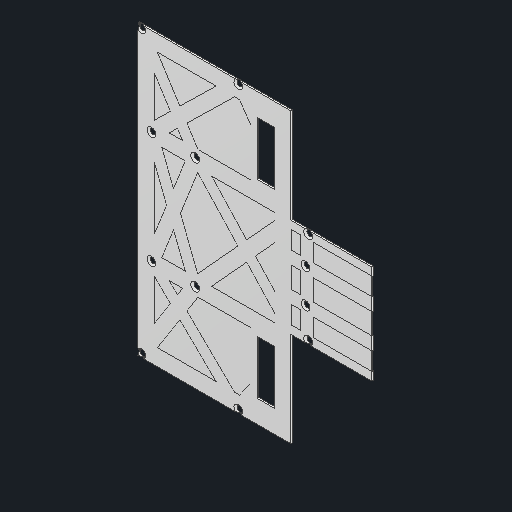
# Autodesk Inventor part: ceil
Saved by Autodesk Inventor 2023 (Build 270158000, 158)
## iProperties
Created: 2024-05-20
Part Number: ceil
Material: ABS Plastic
Document SubType Name: Modeling
Designer: szymo
Density: 1.06 g/cm^3
Appearance: Smooth - White
Mass: 13.9747 g
Surface Area: 401.437 cm^2
Volume: 13.1837 cm^3
Author: szymo
Autodesk Inventor part; units mm, degrees
ref_plane "YZ Plane" through (0, 0, 0) normal (1, 0, 0) x (0, 1, 0)
ref_plane "XZ Plane" through (0, 0, 0) normal (0, 1, 0) x (-1, 0, 0)
ref_plane "XY Plane" through (0, 0, 0) normal (0, 0, 1) x (1, 0, 0)
sketch "Sketch1" plane through (0, 0, 0) normal (0, 0, 1) x (1, 0, 0)
  arc A0 (-30.366, -174.5) -> (-31.2321, -174) centre (-31.2321, -175) ccw
  line L0 (-31.2321, -174) -> (-33.7679, -174)
  arc A1 (-33.7679, -174) -> (-34.634, -174.5) centre (-33.7679, -175) ccw
  arc A2 (-35.5, -175) -> (-34.634, -174.5) centre (-35.5, -174) ccw
  line L1 (-35.5, -175) -> (-89.4385, -175)
  arc A3 (-90.3045, -174.5) -> (-89.4385, -175) centre (-89.4385, -174) ccw
  arc A4 (-90.3045, -174.5) -> (-91.1706, -174) centre (-91.1706, -175) ccw
  line L2 (-91.1706, -174) -> (-93.7065, -174)
  arc A5 (-93.7065, -174) -> (-94.4385, -174.3187) centre (-93.7065, -175) ccw
  line L3 (-94.4385, -178) -> (-94.4385, -174.3187)
  line L4 (-94.4385, -178) -> (0, -178)
  line L5 (0, -178) -> (0, -175)
  line L6 (0, -175) -> (-29.5, -175)
  arc A6 (-30.366, -174.5) -> (-29.5, -175) centre (-29.5, -174) ccw
  circle A7 centre (-92.4385, -176) radius 1.75
  circle A8 centre (-32.5, -176) radius 1.75
  arc A9 (-31.2321, -4) -> (-30.366, -3.5) centre (-31.2321, -3) ccw
  arc A10 (-29.5, -3) -> (-30.366, -3.5) centre (-29.5, -4) ccw
  line L7 (0, -3) -> (-29.5, -3)
  line L8 (0, 0) -> (0, -3)
  line L9 (-94.4385, 0) -> (0, 0)
  line L10 (-94.4385, 0) -> (-94.4385, -3.6813)
  arc A11 (-94.4385, -3.6813) -> (-93.7065, -4) centre (-93.7065, -3) ccw
  line L11 (-91.1706, -4) -> (-93.7065, -4)
  arc A12 (-91.1706, -4) -> (-90.3045, -3.5) centre (-91.1706, -3) ccw
  arc A13 (-89.4385, -3) -> (-90.3045, -3.5) centre (-89.4385, -4) ccw
  line L12 (-35.5, -3) -> (-89.4385, -3)
  arc A14 (-34.634, -3.5) -> (-35.5, -3) centre (-35.5, -4) ccw
  arc A15 (-34.634, -3.5) -> (-33.7679, -4) centre (-33.7679, -3) ccw
  line L13 (-31.2321, -4) -> (-33.7679, -4)
  circle A16 centre (-92.4385, -2) radius 1.75
  circle A17 centre (-32.5, -2) radius 1.75
  circle A18 centre (-59.1371, -54.5) radius 1.75
  circle A19 centre (-86.1669, -54.5) radius 1.75
  spline S0 degree 2 poles (-1.1972, -52) (-3, -52.9286) (-4.8028, -52) knots 0 0 0 1 1 1 weights 1 1.166667 1
  line L14 (-25.1972, -52) -> (-4.8028, -52)
  spline S1 degree 2 poles (-25.1972, -52) (-27, -52.9286) (-28.8028, -52) knots 0 0 0 1 1 1 weights 1 1.166667 1
  line L15 (-94.4385, -52) -> (-28.8028, -52)
  line L16 (-94.4385, -52) -> (-94.4385, -57)
  line L17 (0, -57) -> (-94.4385, -57)
  line L18 (0, -52) -> (0, -57)
  line L19 (-1.1972, -52) -> (0, -52)
  circle A20 centre (-59.1371, -123.5) radius 1.75
  circle A21 centre (-86.1669, -123.5) radius 1.75
  spline S2 degree 2 poles (-1.1972, -126) (-3, -125.0714) (-4.8028, -126) knots 0 0 0 1 1 1 weights 1 1.166667 1
  line L20 (-1.1972, -126) -> (0, -126)
  line L21 (0, -126) -> (0, -121)
  line L22 (0, -121) -> (-94.4385, -121)
  line L23 (-94.4385, -126) -> (-94.4385, -121)
  line L24 (-94.4385, -126) -> (-28.8028, -126)
  spline S3 degree 2 poles (-25.1972, -126) (-27, -125.0714) (-28.8028, -126) knots 0 0 0 1 1 1 weights 1 1.166667 1
  line L25 (-25.1972, -126) -> (-4.8028, -126)
  circle A22 centre (10.6679, -117.5) radius 1.75
  arc A23 (45.504, -115.5) -> (44.7587, -115.8333) centre (45.504, -116.5) ccw
  arc A24 (43.2679, -116.5) -> (44.7587, -115.8333) centre (43.2679, -114.5) ccw
  line L26 (43.2679, -116.5) -> (13.6679, -116.5)
  arc A25 (12.8019, -116) -> (13.6679, -116.5) centre (13.6679, -115.5) ccw
  arc A26 (12.8019, -116) -> (11.9359, -115.5) centre (11.9359, -116.5) ccw
  line L27 (9.4, -115.5) -> (11.9359, -115.5)
  arc A27 (9.4, -115.5) -> (8.534, -116) centre (9.4, -116.5) ccw
  arc A28 (7.6679, -116.5) -> (8.534, -116) centre (7.6679, -115.5) ccw
  line L28 (7.6679, -116.5) -> (-29, -116.5)
  line L29 (-29, -119.5) -> (-29, -116.5)
  line L30 (50, -119.5) -> (-29, -119.5)
  line L31 (50, -119.5) -> (50, -115.5)
  line L32 (50, -115.5) -> (45.504, -115.5)
  line L33 (44, -97.5) -> (44, -101.5)
  line L34 (-29, -97.5) -> (44, -97.5)
  line L35 (-29, -97.5) -> (-29, -101.5)
  line L36 (-29, -101.5) -> (44, -101.5)
  circle A29 centre (8.9832, -99.5) radius 1.75
  line L37 (44, -80.5) -> (44, -76.5)
  line L38 (-29, -76.5) -> (44, -76.5)
  line L39 (-29, -80.5) -> (-29, -76.5)
  line L40 (-29, -80.5) -> (44, -80.5)
  circle A30 centre (8.9832, -78.5) radius 1.75
  circle A31 centre (10.6679, -60.5) radius 1.75
  arc A32 (44.7587, -62.1667) -> (45.504, -62.5) centre (45.504, -61.5) ccw
  line L41 (50, -62.5) -> (45.504, -62.5)
  line L42 (50, -58.5) -> (50, -62.5)
  line L43 (50, -58.5) -> (-29, -58.5)
  line L44 (-29, -58.5) -> (-29, -61.5)
  line L45 (7.6679, -61.5) -> (-29, -61.5)
  arc A33 (8.534, -62) -> (7.6679, -61.5) centre (7.6679, -62.5) ccw
  arc A34 (8.534, -62) -> (9.4, -62.5) centre (9.4, -61.5) ccw
  line L46 (9.4, -62.5) -> (11.9359, -62.5)
  arc A35 (11.9359, -62.5) -> (12.8019, -62) centre (11.9359, -61.5) ccw
  arc A36 (13.6679, -61.5) -> (12.8019, -62) centre (13.6679, -62.5) ccw
  line L47 (43.2679, -61.5) -> (13.6679, -61.5)
  arc A37 (44.7587, -62.1667) -> (43.2679, -61.5) centre (43.2679, -63.5) ccw
  line L48 (0, 0) -> (-94.4385, 0)
  line L49 (-94.4385, 0) -> (-94.4385, -178)
  line L50 (-94.4385, -178) -> (0, -178)
  line L51 (0, -178) -> (0, 0)
  line L52 (0, -58.5) -> (50, -58.5)
  line L53 (50, -58.5) -> (50, -119.5)
  line L54 (50, -119.5) -> (0, -119.5)
  line L55 (0, -119.5) -> (0, -58.5)
  line L56 (0, 0) -> (-94.4385, 0)
  line L57 (-94.4385, 0) -> (-94.4385, -10)
  line L58 (-94.4385, -10) -> (0, -10)
  line L59 (0, -10) -> (0, 0)
  line L60 (-94.4385, -178) -> (0, -178)
  line L61 (0, -178) -> (0, -168)
  line L62 (0, -168) -> (-94.4385, -168)
  line L63 (-94.4385, -168) -> (-94.4385, -178)
  line L64 (-94.4385, -128.5) -> (0, -128.5)
  line L65 (0, -128.5) -> (0, -118.5)
  line L66 (0, -118.5) -> (-94.4385, -118.5)
  line L67 (-94.4385, -118.5) -> (-94.4385, -128.5)
  line L68 (0, -49.5) -> (-94.4385, -49.5)
  line L69 (-94.4385, -49.5) -> (-94.4385, -59.5)
  line L70 (-94.4385, -59.5) -> (0, -59.5)
  line L71 (0, -59.5) -> (0, -49.5)
  line L72 (-94.4385, 0) -> (-84.4385, 0)
  line L73 (-84.4385, 0) -> (-84.4385, -178)
  line L74 (-84.4385, -178) -> (-94.4385, -178)
  line L75 (-94.4385, -178) -> (-94.4385, 0)
  line L76 (0, -178) -> (-10, -178)
  line L77 (-10, -178) -> (-10, 0)
  line L78 (-10, 0) -> (0, 0)
  line L79 (0, 0) -> (0, -178)
  line L80 (0, -58.5) -> (50, -58.5)
  line L81 (50, -58.5) -> (50, -63.5)
  line L82 (50, -63.5) -> (0, -63.5)
  line L83 (0, -63.5) -> (0, -58.5)
  line L84 (0, -119.5) -> (50, -119.5)
  line L85 (50, -119.5) -> (50, -114.5)
  line L86 (50, -114.5) -> (0, -114.5)
  line L87 (0, -114.5) -> (0, -119.5)
  line L88 (0, -74.5) -> (50, -74.5)
  line L89 (50, -74.5) -> (50, -82.5)
  line L90 (50, -82.5) -> (0, -82.5)
  line L91 (0, -82.5) -> (0, -74.5)
  line L92 (0, -95.5) -> (50, -95.5)
  line L93 (50, -95.5) -> (50, -103.5)
  line L94 (50, -103.5) -> (0, -103.5)
  line L95 (0, -103.5) -> (0, -95.5)
  line L96 (13.6679, -58.5) -> (5.6679, -58.5)
  line L97 (5.6679, -58.5) -> (5.6679, -119.5)
  line L98 (5.6679, -119.5) -> (13.6679, -119.5)
  line L99 (13.6679, -119.5) -> (13.6679, -58.5)
  line L100 (-86.1669, -54.5) -> (-32.5, -2) construction
  line L101 (-59.1371, -54.5) -> (-92.4385, -2) construction
  line L102 (-59.1371, -123.5) -> (-92.4385, -176) construction
  line L103 (-32.5, -176) -> (-86.1669, -123.5) construction
  line L104 (-59.1371, -54.5) -> (-86.1669, -123.5) construction
  line L105 (-59.1371, -123.5) -> (-86.1669, -54.5) construction
  line L106 (-32.5, -2) -> (0, -49.5) construction
  line L107 (-32.5, -176) -> (0, -128.5) construction
  line L108 (-59.1371, -54.5) -> (0, -118.5) construction
  line L109 (-59.1371, -123.5) -> (0, -58.5) construction
  line L110 (-22.1796, -10) -> (-10, -27.801)
  line L111 (-10, -41.9682) -> (-31.873, -10)
  line L112 (-84.4385, -47.2135) -> (-46.3979, -10)
  line L113 (-82.6272, -10) -> (-57.5719, -49.5)
  line L114 (-67.0455, -49.5) -> (-84.4385, -22.0798)
  line L115 (-34.9578, -10) -> (-75.3357, -49.5)
  line L116 (-10, -63.5475) -> (-59.9959, -118.5)
  line L117 (-10, -101.7837) -> (-49.0709, -59.5)
  line L118 (-59.9632, -59.5) -> (-9.4803, -114.1342)
  line L119 (-56.7998, -59.5) -> (-79.9123, -118.5)
  line L120 (-56.7998, -118.5) -> (-79.9123, -59.5)
  line L121 (-65.3918, -59.5) -> (-84.4385, -108.1213)
  line L122 (-65.3918, -118.5) -> (-84.4385, -69.8787)
  line L123 (-10, -75.4353) -> (-49.1804, -118.5)
  line L124 (-10, -136.0318) -> (-31.873, -168)
  line L125 (-34.9578, -168) -> (-75.3357, -128.5)
  line L126 (-86.7759, -128.5) -> (-45.3812, -168.9946)
  line L127 (-57.5719, -128.5) -> (-82.6272, -168)
  line L128 (-84.4385, -155.9202) -> (-67.0455, -128.5)
  line L129 (-22.1796, -168) -> (-10, -150.199)
  line L130 (-20.8852, -131) -> (-15.5, -131)
  line L131 (-15.5, -131) -> (-10.1148, -131)
  line L132 (-10.1148, -131) -> (-10.1148, -158.7)
  line L133 (-10.1148, -158.7) -> (-20.8852, -158.7)
  line L134 (-20.8852, -158.7) -> (-20.8852, -131)
  line L135 (-10.1148, -47) -> (-15.5, -47)
  line L136 (-15.5, -47) -> (-20.8852, -47)
  line L137 (-20.8852, -47) -> (-20.8852, -19.3)
  line L138 (-20.8852, -19.3) -> (-10.1148, -19.3)
  line L139 (-10.1148, -19.3) -> (-10.1148, -47)
  line L140 (-24.7852, -157.6409) -> (-24.7852, -128.5)
  line L141 (-24.7852, -20.3591) -> (-24.7852, -49.5)
  line L142 (-19.3, -164.1) -> (-11.7, -164.1)
  line L143 (-19.5112, -164.1) -> (-10, -164.1)
  line L144 (-11.7, -13.9) -> (-19.3, -13.9)
  line L145 (-19.5112, -13.9) -> (-10, -13.9)
  line L146 (-20.8852, -19.3) -> (-20.8852, -10)
  line L147 (-19.5112, -13.9) -> (-20.8852, -13.9)
  line L148 (-20.8852, -158.7) -> (-20.8852, -168)
  line L149 (-19.5112, -164.1) -> (-20.8852, -164.1)
  line L150 (-10.1148, -19.3) -> (-10.1148, -13.9)
  line L151 (-10.1148, -158.7) -> (-10.1148, -164.1)
  point P0 (-15.5, -126)
  point P1 (-15.5, -52)
  point P2 (-17.8691, -161.7)
  point P3 (-10, -161.7)
  point P4 (-17.8691, -16.3)
  point P5 (-10, -16.3)
  point P6 (-27.4828, -94.6513)
  point P7 (-10, -113.5717)
  point P8 (-10, -118.5)
  point P9 (-10, -59.5)
  point P10 (-27.5285, -82.8138)
  point P11 (-64.3739, -38.7765)
  point P12 (-70.22, -44.4955)
  point P13 (-68.7545, -31.8705)
  point P14 (-74.6006, -37.5894)
  point P15 (-10, -10)
  point P16 (-10.1148, -41.8004)
  point P17 (-10.1148, -27.6332)
  point P18 (5.6679, -114.5)
  point P19 (0, -114.5)
  point P20 (0, -103.5)
  point P21 (5.6679, -103.5)
  point P22 (5.6679, -74.5)
  point P23 (0, -63.5)
  point P24 (5.6679, -63.5)
  point P25 (-72.652, -99.9665)
  point P26 (-76.948, -89)
  point P27 (-57.7417, -61.9042)
  point P28 (-32.9325, -88.7535)
  point P29 (-57.7618, -116.0444)
  point P30 (-68.3561, -89)
  point P31 (-46.3979, -168)
  point P32 (-68.7545, -146.1295)
  point P33 (-84.4385, -130.7865)
  point P34 (-74.6006, -140.4106)
  point P35 (-70.22, -133.5045)
  point P36 (-10.1148, -150.3668)
  point P37 (-10.1148, -136.1996)
  point P38 (-64.3739, -139.2235)
  point P39 (-72.652, -78.0335)
  point P40 (-22.0788, -88.7116)
  point P41 (5.6679, -95.5)
  point P42 (0, -82.5)
  point P43 (5.6679, -82.5)
  point P44 (-10, -168)
  point P45 (-94.4385, -52.0054)
  point P46 (13.6679, -114.5)
  point P47 (13.6679, -103.5)
  point P48 (13.6679, -95.5)
  point P49 (13.6679, -82.5)
  point P50 (13.6679, -74.5)
  point P51 (13.6679, -63.5)
  point P52 (-10, 0)
  point P53 (-20.8852, -151.9409)
  dimension "d0" = 10
  dimension "d1" = 10
  dimension "d2" = 5
  dimension "d3" = 5
  dimension "d4" = 5
  dimension "d5" = 5
  dimension "d6" = 10
  dimension "d7" = 10
  dimension "d8" = 5
  dimension "d9" = 5
  dimension "d10" = 4
  dimension "d11" = 4
  dimension "d12" = 4
  dimension "d13" = 4
  dimension "d14" = 3
  dimension "d15" = 5
  dimension "d16" = 4
  dimension "d17" = 4
  dimension "d18" = 4
  dimension "d19" = 4
  dimension "d20" = 4
  dimension "d21" = 4
  dimension "d22" = 4
  dimension "d23" = 4
  dimension "d24" = 4
  dimension "d25" = 4
  dimension "d26" = 4
  dimension "d27" = 4
  dimension "d28" = 4
  dimension "d29" = 4
  dimension "d30" = 4
  dimension "d31" = 4
  dimension "d32" = 4
  dimension "d33" = 4
  dimension "d34" = 4
  dimension "d35" = 4
  dimension "d37" = 3.9
  dimension "d39" = 3.9
  dimension "d42" = 3.9
  dimension "d44" = 3.9
  constraints: 202 end point, 66 point on line, 45 parallel, 21 horizontal, 18 perpendicular, 5 vertical, 2 collinear, 24 other
  measures "d0" distance of L57.end L56.end
  measures "d1" distance of L61.end L60.end
  measures "d2" distance from line of L101.start L70
  measures "d3" distance from line of L68 L101.start
  measures "d4" distance from line of L66 L102.start
  measures "d5" distance from line of L64 L102.start
  measures "d6" distance of L73.end L74.end
  measures "d7" distance of L78.start L78.end
  measures "d8" distance between parallel lines of L52 L82
  measures "d9" distance between parallel lines of L86 L84
  measures "d10" distance from line of A30.centre L90
  measures "d11" distance from line of A30.centre L88
  measures "d12" distance from line of A29.centre L92
  measures "d13" distance from line of A29.centre L94
  measures "d14" distance from line of L99 A31.centre
  measures "d15" distance from line of A31.centre L97
  measures "d16" distance between parallel lines of L106 L111
  measures "d17" distance between parallel lines of L110 L106
  measures "d18" distance between parallel lines of L100 L115
  measures "d19" distance between parallel lines of L100 L112
  measures "d20" distance between parallel lines of L101 L113
  measures "d21" distance between parallel lines of L101 L114
  measures "d22" distance between parallel lines of L108 L118
  measures "d23" distance between parallel lines of L108 L117
  measures "d24" distance between parallel lines of L109 L123
  measures "d25" distance between parallel lines of L109 L116
  measures "d26" distance between parallel lines of L105 L120
  measures "d27" distance between parallel lines of L105 L122
  measures "d28" distance between parallel lines of L104 L119
  measures "d29" distance between parallel lines of L104 L121
  measures "d30" distance between parallel lines of L125 L103
  measures "d31" distance between parallel lines of L126 L103
  measures "d32" distance between parallel lines of L102 L127
  measures "d33" distance between parallel lines of L102 L128
  measures "d34" distance between parallel lines of L107 L124
  measures "d35" distance between parallel lines of L107 L129
  measures "d37" distance between parallel lines of L134 L140
  measures "d39" distance between parallel lines of L137 L141
  measures "d42" distance between parallel lines of L62 L142
  measures "d44" distance between parallel lines of L58 L144
extrude "Extrusion1" add sketch "Sketch1" along normal blind 0.8 contours A6 L6 L77 L4 L73 L1 A2 A1 L0 A0 | A0 L0 A1 A2 L1 L73 L62 L77 L6 A6 | L77 L62 L51 L6 | L6 L5 L4 L77 | L77 L64 L51 L62 | L62 L148 L129 L143 L142 L77 | L4 L3 A5 L2 A4 A3 L1 L73 | L62 L129 L148 | L143 L151 L132 L129 L77 | L1 A3 A4 L2 A5 L49 L62 L73 | L64 L77 L25 S2 L20 L51 | L62 L124 L134 L148 L129 | L148 L149 L129 | L129 L132 L124 L77 | L73 L128 L126 L127 L62 | L62 L49 L64 L126 L73 | L20 S2 L25 L77 L22 L21 | L77 L124 L132 L131 L130 L134 L140 L64 | L64 L73 L24 S3 L25 L77 | L22 L77 L30 L51 | L25 S3 L24 L73 A21 L22 L77 | L62 L126 L127 L125 | L126 L128 L125 L127 | L49 L24 L73 L64 | L126 L64 L73 | L73 L64 L125 L128 L126 | L22 L73 L66 L29 L30 L77 | L51 L28 L97 L30 | L30 L77 L66 L51 | L127 L125 L128 L64 | L23 L22 L73 A21 L24 | L22 L49 L66 L73 | L30 L29 L66 L77 | L97 L28 A28 A27 L27 A26 A25 L99 L30 | L66 L77 L28 L51 | L73 L121 L122 L119 L66 | L66 L49 L70 L73 | L73 A21 | A21 L73 | L99 L26 A24 A23 L32 L31 L30 | L97 L86 L99 A25 A26 L27 A27 A28 L28 | L28 L51 L86 L97 | L28 L77 L36 L51 | L99 L86 L53 L32 A23 A24 L26 | L97 L94 L99 L86 | L49 L17 L73 L70 | L122 L119 L120 L116 L66 | L122 L121 L120 L119 | L73 L70 L120 L121 L122 | L66 L120 L116 L118 L123 | L118 L36 L117 L77 | L97 L36 L99 L94 | L94 L51 L36 L97 | L16 L15 L73 A19 L17 | L73 L17 L77 L43 L44 L70 | L116 L120 L66 | L120 L121 L70 L118 L119 | L123 L117 L34 L118 | L118 L116 L117 L123 | L118 L34 L117 L36 | L99 L36 L33 L34 L92 L53 L94 | L97 L34 L99 L36 | L36 L51 L34 L97 | L36 L77 L34 L51 | L49 L68 L73 L15 | L73 A19 L15 S1 L14 L77 L17 | L119 L70 L117 L116 L118 | L118 L70 L119 | L117 L116 L40 L123 | L99 L34 L33 L36 | L97 L92 L99 L34 | L34 L51 L92 L97 | L34 L77 L40 L51 | L73 L68 L77 L14 S1 L15 | L49 L58 L73 L68 | L77 L14 S0 L19 L18 L17 | L17 L51 L43 L77 | L73 A19 | A19 L73 | L40 L116 L38 L123 | L97 L90 L99 L92 | L73 L112 L114 L115 L68 | L49 A11 L11 A12 A13 L12 L73 L58 | L77 L70 L44 L43 | L43 L51 L70 L77 | L77 L68 L51 L19 S0 L14 | L77 L38 L51 L40 | L38 L116 L77 L123 | L90 L99 L40 L37 L38 L88 L53 | L97 L40 L99 L90 | L90 L51 L40 L97 | L10 L9 L73 L12 A13 A12 L11 A11 | L73 L12 A14 A15 L13 A9 A10 L7 L77 L58 | L58 L113 L112 L114 L73 | L43 L97 L45 L51 | L70 L51 L45 L77 | L77 L58 L51 L68 | L68 L141 L111 L137 L136 L135 L139 L77 | L51 L38 L97 L40 | L77 L45 L51 L38 | L97 L38 L99 L40 | L114 L115 L113 L68 | L114 L112 L113 L115 | L73 L9 L77 L7 A10 A9 L13 A15 A14 L12 | L43 L99 A36 A35 L46 A34 A33 L45 L97 | L111 L139 L110 L77 | L51 L88 L97 L38 | L82 L99 L47 A37 A32 L41 L53 | L99 L38 L97 L88 | L88 L97 L82 L99 | L99 L38 L37 L40 | L113 L112 L58 L115 | L58 L77 L7 L51 | L43 L42 L41 A32 A37 L47 L99 | L97 L82 L51 L45 | L45 A33 A34 L46 A35 A36 L99 L82 L97 | L111 L58 L110 L146 L137 | L110 L139 L150 L145 L77 | L9 L8 L7 L77 | L77 L145 L144 L110 L146 L58 | L146 L110 L58 | L110 L147 L146 | A7 | A8 | A16 | A17 | A18 | A20 | A22 | A29 | A30 | A31
sketch "Sketch3" plane through (0, 0, 0.8) normal (0, 0, 1) x (1, 0, 0)
  line L0 (-94.4385, 0) -> (-94.4385, -178) projected
  line L1 (-94.4385, -178) -> (0, -178) projected
  line L2 (0, -178) -> (0, -119.5) projected
  line L3 (0, -119.5) -> (50, -119.5) projected
  line L4 (50, -119.5) -> (50, -114.5) projected
  line L5 (50, -114.5) -> (13.6679, -114.5) projected
  line L6 (13.6679, -114.5) -> (13.6679, -103.5) projected
  line L7 (13.6679, -103.5) -> (50, -103.5) projected
  line L8 (50, -103.5) -> (50, -95.5) projected
  line L9 (50, -95.5) -> (13.6679, -95.5) projected
  line L10 (13.6679, -95.5) -> (13.6679, -82.5) projected
  line L11 (13.6679, -82.5) -> (50, -82.5) projected
  line L12 (50, -82.5) -> (50, -74.5) projected
  line L13 (50, -74.5) -> (13.6679, -74.5) projected
  line L14 (13.6679, -74.5) -> (13.6679, -63.5) projected
  line L15 (13.6679, -63.5) -> (50, -63.5) projected
  line L16 (50, -63.5) -> (50, -58.5) projected
  line L17 (50, -58.5) -> (0, -58.5) projected
  line L18 (0, -58.5) -> (0, 0) projected
  line L19 (0, 0) -> (-94.4385, 0) projected
  line L20 (-10, -118.5) -> (-49.1804, -118.5) projected
  line L21 (-49.1804, -118.5) -> (-27.4828, -94.6513) projected
  line L22 (-27.4828, -94.6513) -> (-10, -113.5717) projected
  line L23 (-10, -113.5717) -> (-10, -118.5) projected
  line L24 (-84.4385, -22.0798) -> (-74.6006, -37.5894) projected
  line L25 (-74.6006, -37.5894) -> (-84.4385, -47.2135) projected
  line L26 (-84.4385, -47.2135) -> (-84.4385, -22.0798) projected
  line L27 (-70.22, -44.4955) -> (-67.0455, -49.5) projected
  line L28 (-67.0455, -49.5) -> (-75.3357, -49.5) projected
  line L29 (-75.3357, -49.5) -> (-70.22, -44.4955) projected
  line L30 (-20.8852, -47) -> (-20.8852, -13.9) projected
  line L31 (-20.8852, -13.9) -> (-10.1148, -13.9) projected
  line L32 (-10.1148, -13.9) -> (-10.1148, -47) projected
  line L33 (-10.1148, -47) -> (-20.8852, -47) projected
  line L34 (-68.7545, -31.8705) -> (-82.6272, -10) projected
  line L35 (-82.6272, -10) -> (-46.3979, -10) projected
  line L36 (-46.3979, -10) -> (-68.7545, -31.8705) projected
  line L37 (-49.0709, -59.5) -> (-10, -59.5) projected
  line L38 (-10, -59.5) -> (-10, -63.5475) projected
  line L39 (-10, -63.5475) -> (-27.5285, -82.8138) projected
  line L40 (-27.5285, -82.8138) -> (-49.0709, -59.5) projected
  line L41 (-24.7852, -20.3591) -> (-24.7852, -49.5) projected
  line L42 (-24.7852, -49.5) -> (-57.5719, -49.5) projected
  line L43 (-57.5719, -49.5) -> (-64.3739, -38.7765) projected
  line L44 (-64.3739, -38.7765) -> (-34.9578, -10) projected
  line L45 (-34.9578, -10) -> (-31.873, -10) projected
  line L46 (-31.873, -10) -> (-24.7852, -20.3591) projected
  line L47 (5.6679, -114.5) -> (0, -114.5) projected
  line L48 (0, -114.5) -> (0, -103.5) projected
  line L49 (0, -103.5) -> (5.6679, -103.5) projected
  line L50 (5.6679, -103.5) -> (5.6679, -114.5) projected
  line L51 (5.6679, -74.5) -> (0, -74.5) projected
  line L52 (0, -74.5) -> (0, -63.5) projected
  line L53 (0, -63.5) -> (5.6679, -63.5) projected
  line L54 (5.6679, -63.5) -> (5.6679, -74.5) projected
  line L55 (-65.3918, -59.5) -> (-72.652, -78.0335) projected
  line L56 (-72.652, -78.0335) -> (-79.9123, -59.5) projected
  line L57 (-79.9123, -59.5) -> (-65.3918, -59.5) projected
  line L58 (-46.3979, -168) -> (-82.6272, -168) projected
  line L59 (-82.6272, -168) -> (-68.7545, -146.1295) projected
  line L60 (-68.7545, -146.1295) -> (-46.3979, -168) projected
  line L61 (-84.4385, -130.7865) -> (-74.6006, -140.4106) projected
  line L62 (-74.6006, -140.4106) -> (-84.4385, -155.9202) projected
  line L63 (-84.4385, -155.9202) -> (-84.4385, -130.7865) projected
  line L64 (-75.3357, -128.5) -> (-67.0455, -128.5) projected
  line L65 (-67.0455, -128.5) -> (-70.22, -133.5045) projected
  line L66 (-70.22, -133.5045) -> (-75.3357, -128.5) projected
  line L67 (-10.1148, -131) -> (-10.1148, -164.1) projected
  line L68 (-10.1148, -164.1) -> (-20.8852, -164.1) projected
  line L69 (-20.8852, -164.1) -> (-20.8852, -131) projected
  line L70 (-20.8852, -131) -> (-10.1148, -131) projected
  line L71 (-34.9578, -168) -> (-64.3739, -139.2235) projected
  line L72 (-64.3739, -139.2235) -> (-57.5719, -128.5) projected
  line L73 (-57.5719, -128.5) -> (-24.7852, -128.5) projected
  line L74 (-24.7852, -128.5) -> (-24.7852, -157.6409) projected
  line L75 (-24.7852, -157.6409) -> (-31.873, -168) projected
  line L76 (-31.873, -168) -> (-34.9578, -168) projected
  line L77 (-32.9325, -88.7535) -> (-57.7618, -116.0444) projected
  line L78 (-57.7618, -116.0444) -> (-68.3561, -89) projected
  line L79 (-68.3561, -89) -> (-57.7417, -61.9042) projected
  line L80 (-57.7417, -61.9042) -> (-32.9325, -88.7535) projected
  line L81 (-84.4385, -108.1213) -> (-84.4385, -69.8787) projected
  line L82 (-84.4385, -69.8787) -> (-76.948, -89) projected
  line L83 (-76.948, -89) -> (-84.4385, -108.1213) projected
  line L84 (-79.9123, -118.5) -> (-72.652, -99.9665) projected
  line L85 (-72.652, -99.9665) -> (-65.3918, -118.5) projected
  line L86 (-65.3918, -118.5) -> (-79.9123, -118.5) projected
  line L87 (-10, -75.4353) -> (-10, -101.7837) projected
  line L88 (-10, -101.7837) -> (-22.0788, -88.7116) projected
  line L89 (-22.0788, -88.7116) -> (-10, -75.4353) projected
  line L90 (5.6679, -95.5) -> (0, -95.5) projected
  line L91 (0, -95.5) -> (0, -82.5) projected
  line L92 (0, -82.5) -> (5.6679, -82.5) projected
  line L93 (5.6679, -82.5) -> (5.6679, -95.5) projected
  line L94 (-94.4385, 0) -> (0, 0)
  line L95 (0, 0) -> (0, -178)
  line L96 (0, -178) -> (-94.4385, -178)
  line L97 (-94.4385, -178) -> (-94.4385, 0)
  line L98 (0, -119.5) -> (50, -119.5)
  line L99 (50, -119.5) -> (50, -58.5)
  line L100 (50, -58.5) -> (0, -58.5)
  line L101 (0, -58.5) -> (0, -119.5)
  constraints: 16 end point, 4 parallel, 2 horizontal, 2 perpendicular
extrude "Extrusion2" add sketch "Sketch3" along normal blind 0.2 contours L19 L18 L95 L52 L91 L48 L2 L1 L0 | L17 L16 L15 L14 L13 L12 L11 L10 L9 L8 L7 L6 L5 L4 L3 L95 L47 L50 L49 L90 L93 L92 L51 L54 L53 | L53 L54 L51 L52 | L48 L49 L50 L47 | L99 L13 L14 L15 | L5 L6 L7 L99 | L92 L93 L90 L91 | L99 L9 L10 L11 | L20 L21 L22 L23 | L24 L25 L26 | L27 L28 L29 | L34 L35 L36 | L37 L38 L39 L40 | L41 L42 L43 L44 L45 L46 | L55 L56 L57 | L58 L59 L60 | L61 L62 L63 | L64 L65 L66 | L71 L72 L73 L74 L75 L76 | L77 L78 L79 L80 | L81 L82 L83 | L84 L85 L86 | L87 L88 L89
sketch "Sketch4" plane through (0, 0, 1) normal (0, 0, 1) x (1, 0, 0)
  circle A0 centre (10.6679, -117.5) radius 1.75
  arc A1 (45.504, -115.5) -> (44.7587, -115.8333) centre (45.504, -116.5) ccw
  arc A2 (43.2679, -116.5) -> (44.7587, -115.8333) centre (43.2679, -114.5) ccw
  line L0 (43.2679, -116.5) -> (13.6679, -116.5)
  arc A3 (12.8019, -116) -> (13.6679, -116.5) centre (13.6679, -115.5) ccw
  arc A4 (12.8019, -116) -> (11.9359, -115.5) centre (11.9359, -116.5) ccw
  line L1 (9.4, -115.5) -> (11.9359, -115.5)
  arc A5 (9.4, -115.5) -> (8.534, -116) centre (9.4, -116.5) ccw
  arc A6 (7.6679, -116.5) -> (8.534, -116) centre (7.6679, -115.5) ccw
  line L2 (7.6679, -116.5) -> (-29, -116.5)
  line L3 (-29, -119.5) -> (-29, -116.5)
  line L4 (50, -119.5) -> (-29, -119.5)
  line L5 (50, -119.5) -> (50, -115.5)
  line L6 (50, -115.5) -> (45.504, -115.5)
  line L7 (44, -97.5) -> (44, -101.5)
  line L8 (-29, -97.5) -> (44, -97.5)
  line L9 (-29, -97.5) -> (-29, -101.5)
  line L10 (-29, -101.5) -> (44, -101.5)
  circle A7 centre (8.9832, -99.5) radius 1.75
  line L11 (44, -80.5) -> (44, -76.5)
  line L12 (-29, -76.5) -> (44, -76.5)
  line L13 (-29, -80.5) -> (-29, -76.5)
  line L14 (-29, -80.5) -> (44, -80.5)
  circle A8 centre (8.9832, -78.5) radius 1.75
  circle A9 centre (10.6679, -60.5) radius 1.75
  arc A10 (44.7587, -62.1667) -> (45.504, -62.5) centre (45.504, -61.5) ccw
  line L15 (50, -62.5) -> (45.504, -62.5)
  line L16 (50, -58.5) -> (50, -62.5)
  line L17 (50, -58.5) -> (-29, -58.5)
  line L18 (-29, -58.5) -> (-29, -61.5)
  line L19 (7.6679, -61.5) -> (-29, -61.5)
  arc A11 (8.534, -62) -> (7.6679, -61.5) centre (7.6679, -62.5) ccw
  arc A12 (8.534, -62) -> (9.4, -62.5) centre (9.4, -61.5) ccw
  line L20 (9.4, -62.5) -> (11.9359, -62.5)
  arc A13 (11.9359, -62.5) -> (12.8019, -62) centre (11.9359, -61.5) ccw
  arc A14 (13.6679, -61.5) -> (12.8019, -62) centre (13.6679, -62.5) ccw
  line L21 (43.2679, -61.5) -> (13.6679, -61.5)
  arc A15 (44.7587, -62.1667) -> (43.2679, -61.5) centre (43.2679, -63.5) ccw
  arc A16 (-30.366, -174.5) -> (-31.2321, -174) centre (-31.2321, -175) ccw
  line L22 (-31.2321, -174) -> (-33.7679, -174)
  arc A17 (-33.7679, -174) -> (-34.634, -174.5) centre (-33.7679, -175) ccw
  arc A18 (-35.5, -175) -> (-34.634, -174.5) centre (-35.5, -174) ccw
  line L23 (-35.5, -175) -> (-89.4385, -175)
  arc A19 (-90.3045, -174.5) -> (-89.4385, -175) centre (-89.4385, -174) ccw
  arc A20 (-90.3045, -174.5) -> (-91.1706, -174) centre (-91.1706, -175) ccw
  line L24 (-91.1706, -174) -> (-93.7065, -174)
  arc A21 (-93.7065, -174) -> (-94.4385, -174.3187) centre (-93.7065, -175) ccw
  line L25 (-94.4385, -178) -> (-94.4385, -174.3187)
  line L26 (-94.4385, -178) -> (0, -178)
  line L27 (0, -178) -> (0, -175)
  line L28 (0, -175) -> (-29.5, -175)
  arc A22 (-30.366, -174.5) -> (-29.5, -175) centre (-29.5, -174) ccw
  circle A23 centre (-92.4385, -176) radius 1.75
  circle A24 centre (-32.5, -176) radius 1.75
  circle A25 centre (-59.1371, -123.5) radius 1.75
  circle A26 centre (-86.1669, -123.5) radius 1.75
  spline S0 degree 2 poles (-1.1972, -126) (-3, -125.0714) (-4.8028, -126) knots 0 0 0 1 1 1 weights 1 1.166667 1
  line L29 (-1.1972, -126) -> (0, -126)
  line L30 (0, -126) -> (0, -121)
  line L31 (0, -121) -> (-94.4385, -121)
  line L32 (-94.4385, -126) -> (-94.4385, -121)
  line L33 (-94.4385, -126) -> (-28.8028, -126)
  spline S1 degree 2 poles (-25.1972, -126) (-27, -125.0714) (-28.8028, -126) knots 0 0 0 1 1 1 weights 1 1.166667 1
  line L34 (-25.1972, -126) -> (-4.8028, -126)
  circle A27 centre (-59.1371, -54.5) radius 1.75
  circle A28 centre (-86.1669, -54.5) radius 1.75
  spline S2 degree 2 poles (-1.1972, -52) (-3, -52.9286) (-4.8028, -52) knots 0 0 0 1 1 1 weights 1 1.166667 1
  line L35 (-25.1972, -52) -> (-4.8028, -52)
  spline S3 degree 2 poles (-25.1972, -52) (-27, -52.9286) (-28.8028, -52) knots 0 0 0 1 1 1 weights 1 1.166667 1
  line L36 (-94.4385, -52) -> (-28.8028, -52)
  line L37 (-94.4385, -52) -> (-94.4385, -57)
  line L38 (0, -57) -> (-94.4385, -57)
  line L39 (0, -52) -> (0, -57)
  line L40 (-1.1972, -52) -> (0, -52)
  arc A29 (-31.2321, -4) -> (-30.366, -3.5) centre (-31.2321, -3) ccw
  arc A30 (-29.5, -3) -> (-30.366, -3.5) centre (-29.5, -4) ccw
  line L41 (0, -3) -> (-29.5, -3)
  line L42 (0, 0) -> (0, -3)
  line L43 (-94.4385, 0) -> (0, 0)
  line L44 (-94.4385, 0) -> (-94.4385, -3.6813)
  arc A31 (-94.4385, -3.6813) -> (-93.7065, -4) centre (-93.7065, -3) ccw
  line L45 (-91.1706, -4) -> (-93.7065, -4)
  arc A32 (-91.1706, -4) -> (-90.3045, -3.5) centre (-91.1706, -3) ccw
  arc A33 (-89.4385, -3) -> (-90.3045, -3.5) centre (-89.4385, -4) ccw
  line L46 (-35.5, -3) -> (-89.4385, -3)
  arc A34 (-34.634, -3.5) -> (-35.5, -3) centre (-35.5, -4) ccw
  arc A35 (-34.634, -3.5) -> (-33.7679, -4) centre (-33.7679, -3) ccw
  line L47 (-31.2321, -4) -> (-33.7679, -4)
  circle A36 centre (-92.4385, -2) radius 1.75
  circle A37 centre (-32.5, -2) radius 1.75
  constraints: 12 coincident
hole "Hole1" at (-32.5, -2, 1) at (-92.4385, -2, 1) at (-86.1669, -54.5, 1) at (-59.1371, -54.5, 1) at (-86.1669, -123.5, 1) at (-59.1371, -123.5, 1) at (-92.4385, -176, 1) at (-32.5, -176, 1) at (10.6679, -60.5, 1) at (8.9832, -78.5, 1) at (8.9832, -99.5, 1) at (10.6679, -117.5, 1) direction (0, 0, -1) diameter 3.1 end through all countersink diameter 5.5 countersink angle 90 clearance for "Countersunk Flat Head Screw ISO 2009/7046" size "M2.5" standard "ISO"
equation "\"d0\" = d7"
equation "\"d1\" = d7"
equation "\"d2\" = 0.5 * d7"
equation "\"d3\" = 0.5 * d7"
equation "\"d4\" = 0.5 * d7"
equation "\"d5\" = 0.5 * d7"
equation "\"d6\" = d7"
equation "\"d8\" = 0.5 * d7"
equation "\"d9\" = 0.5 * d7"
equation "\"d15\" = 0.5 * d7"
equation "\"d18\" = d17"
equation "\"d19\" = d17"
equation "\"d20\" = d17"
equation "\"d21\" = d17"
equation "\"d22\" = d17"
equation "\"d23\" = d17"
equation "\"d24\" = d17"
equation "\"d25\" = d17"
equation "\"d26\" = d17"
equation "\"d27\" = d17"
equation "\"d28\" = d17"
equation "\"d29\" = d17"
equation "\"d30\" = d17"
equation "\"d31\" = d17"
equation "\"d32\" = d17"
equation "\"d33\" = d17"
equation "\"d34\" = d17"
equation "\"d35\" = d17"
body "Solid1"
